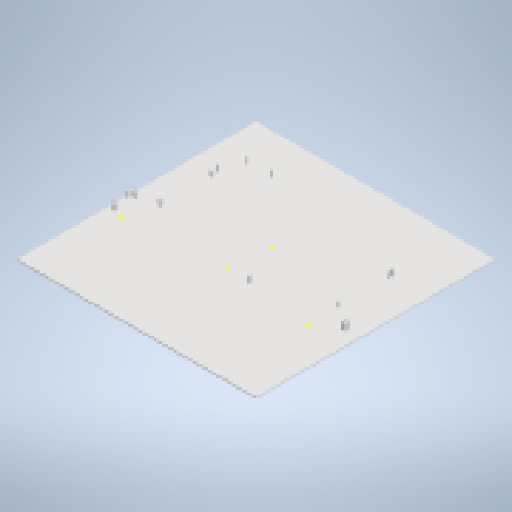
# Autodesk Inventor part: chassis
Saved by Autodesk Inventor 2025 (Build 290162010, 162A)
## iProperties
Created: 2025-12-11
Part Number: chassis
Material: Generic
Document SubType Name: Modeling
Designer: 200481997
Density: 1 g/cm^3
Appearance: Default
Author: 200481997
Autodesk Inventor part; units mm, degrees
ref_plane "YZ Plane" through (0, 0, 0) normal (1, 0, 0) x (0, 1, 0)
ref_plane "XZ Plane" through (0, 0, 0) normal (0, 1, 0) x (-1, 0, 0)
ref_plane "XY Plane" through (0, 0, 0) normal (0, 0, 1) x (1, 0, 0)
sketch "Sketch3" plane through (0, 0, 0) normal (0, 1, 0) x (-1, 0, 0)
  line L0 (-150, -128.5714) -> (150, -128.5714)
  line L1 (150, -128.5714) -> (150, 171.4286)
  line L2 (150, 171.4286) -> (-150, 171.4286)
  line L3 (-150, 171.4286) -> (-150, -128.5714)
  point P0 (0, 0)
  dimension "d80" = 300
  dimension "d81" = 300
  dimension "d82" = 150
  dimension "d83" = 128.5714
  constraints: 8 end point, 2 parallel, 1 horizontal, 1 perpendicular
  measures "d80" distance between parallel lines of L2 L0
  measures "d81" distance between parallel lines of L1 L3
  measures "d82" distance from line of point (0, 0) L3
  measures "d83" distance from line of point (0, 0) L0
extrude "Chassis base" add sketch "Sketch3" against normal blind 1.5875
sketch "Motherboard Mounting Holes" plane through (0, 0, 0) normal (0, 1, 0) x (-1, 0, 0)
  circle A0 centre (142.65, 56.4682) radius 1.15
  circle A1 centre (142.65, 56.4682) radius 2.5
  circle A2 centre (118.8, -41.6318) radius 2.05
  circle A3 centre (143.65, 30.0682) radius 1.15
  circle A4 centre (142.65, 56.4682) radius 2.5
  circle A5 centre (118.8, -41.6318) radius 0.7
  circle A6 centre (143.65, 30.0682) radius 2.5
  circle A7 centre (148.65, 51.0682) radius 1.1
  circle A8 centre (118.8, 22.3682) radius 0.7
  circle A9 centre (118.8, -41.6318) radius 2.05
  circle A10 centre (148.65, 34.0682) radius 1.1
  circle A11 centre (119.95, -50.0818) radius 1.25
  circle A12 centre (-102.85, -46.4318) radius 2
  circle A13 centre (-102.85, -46.4318) radius 0.9
  circle A14 centre (-103.35, 21.2682) radius 1.85
  circle A15 centre (-131, 40.4962) radius 4
  circle A16 centre (-103.35, 21.2682) radius 0.9
  circle A17 centre (-131, 40.4962) radius 1.35
  circle A18 centre (-103.35, -41.5818) radius 1.25
  circle A19 centre (-20.85, 50.0682) radius 0.9
  circle A20 centre (118.8, 22.3682) radius 2.05
  circle A21 centre (-20.85, 50.0682) radius 2
  circle A22 centre (118.8, -41.6318) radius 2.05
  circle A23 centre (142.65, 56.4682) radius 2.5
  circle A24 centre (118.8, -41.6318) radius 2.05
  circle A25 centre (148.65, 51.0682) radius 1.8
  circle A26 centre (148.65, 34.0682) radius 1.8
  line L0 (119.55, -51.2661) -> (119.55, -48.8975)
  line L1 (120.35, -48.8975) -> (120.35, -51.2661)
  line L2 (120.35, -51.6947) -> (119.55, -48.4689) construction
  line L3 (119.55, -51.6947) -> (120.35, -48.4689) construction
  line L4 (121.1343, -49.6818) -> (118.7657, -49.6818)
  line L5 (118.7657, -50.4818) -> (121.1343, -50.4818)
  line L6 (122.1914, -49.6818) -> (117.7086, -50.4818) construction
  line L7 (117.7086, -49.6818) -> (122.1914, -50.4818) construction
  line L8 (-103.75, -42.7661) -> (-103.75, -40.3975)
  line L9 (-102.95, -40.3975) -> (-102.95, -42.7661)
  line L10 (-102.95, -43.2946) -> (-103.75, -39.869) construction
  line L11 (-103.75, -43.2946) -> (-102.95, -39.869) construction
  line L12 (-102.1657, -41.1818) -> (-104.5343, -41.1818)
  line L13 (-104.5343, -41.9818) -> (-102.1657, -41.9818)
  line L14 (-101.5, -41.1818) -> (-105.2, -41.9818) construction
  line L15 (-105.2, -41.1818) -> (-101.5, -41.9818) construction
  point P0 (0, 0)
  point P1 (-102.95, -41.1818)
  point P2 (-103.75, -41.1818)
  point P3 (-103.75, -41.9818)
  point P4 (-102.95, -41.9818)
  point P5 (119.55, -50.4818)
  point P6 (120.35, -50.4818)
  point P7 (120.35, -49.6818)
  point P8 (119.55, -49.6818)
  dimension "d12" = 2.5
  dimension "d39" = 2.5
  dimension "d0" = 41.6318
  dimension "d1" = 118.8
  dimension "d2" = 8.45
  dimension "d3" = 1.15
  dimension "d8" = 102.85
  dimension "d9" = 46.4318
  dimension "d10" = 1.8
  dimension "d11" = 4
  dimension "d13" = 4.85
  dimension "d14" = 0.5
  dimension "d15" = 50.0682
  dimension "d16" = 20.85
  dimension "d17" = 1.8
  dimension "d18" = 4
  dimension "d19" = 103.35
  dimension "d20" = 21.2682
  dimension "d21" = 1.8
  dimension "d22" = 3.7
  dimension "d23" = 118.8
  dimension "d24" = 22.3682
  dimension "d25" = 1.4
  dimension "d26" = 4.1
  dimension "d27" = 143.65
  dimension "d28" = 30.0682
  dimension "d29" = 2.3
  dimension "d30" = 5
  dimension "d31" = 4
  dimension "d32" = 5
  dimension "d33" = 2.2
  dimension "d34" = 3.6
  dimension "d35" = 17
  dimension "d36" = 5.4
  dimension "d37" = 1.4
  dimension "d38" = 4.1
  dimension "d40" = 131
  dimension "d41" = 40.4962
  dimension "d42" = 6
  dimension "d52" = 8
  dimension "d53" = 2.7
  dimension "d66" = 0.8
  dimension "d67" = 0.8
  dimension "d68" = 0.8
  dimension "d69" = 0.8
  dimension "d71" = 0.4
  dimension "d72" = 0.4
  dimension "d73" = 0.4
  dimension "d74" = 0.4
  constraints: 32 end point, 25 centre point, 10 concentric, 8 midpoint, 4 equal radius, 4 parallel, 2 horizontal, 1 vertical alignment, 20 other
  measures "d0" vertical distance of point (0, 0) A2.centre
  measures "d1" horizontal distance of point (0, 0) A2.centre
  measures "d2" vertical distance of A2.centre point (119.95, -50.082)
  measures "d3" horizontal distance of point (119.95, -50.082) A2.centre
  measures "d8" horizontal distance of point (0, 0) A12.centre
  measures "d9" vertical distance of point (0, 0) A12.centre
  measures "d10" diameter of A13
  measures "d11" diameter of A12
  measures "d13" vertical distance of point (-103.35, -41.582) A12.centre
  measures "d14" horizontal distance of A12.centre point (-103.35, -41.582)
  measures "d15" vertical distance of point (0, 0) A19.centre
  measures "d16" horizontal distance of point (0, 0) A19.centre
  measures "d17" diameter of A19
  measures "d18" diameter of A21
  measures "d19" horizontal distance of point (0, 0) A14.centre
  measures "d20" vertical distance of A14.centre point (0, 0)
  measures "d21" diameter of A16
  measures "d22" diameter of A14
  measures "d23" horizontal distance of point (0, 0) A8.centre
  measures "d24" vertical distance of point (0, 0) A8.centre
  measures "d25" diameter of A8
  measures "d26" diameter of A20
  measures "d27" horizontal distance of point (0, 0) A3.centre
  measures "d28" vertical distance of point (0, 0) A3.centre
  measures "d29" diameter of A3
  measures "d30" diameter of A6
  measures "d31" vertical distance of A3.centre A10.centre
  measures "d32" horizontal distance of A3.centre A10.centre
  measures "d33" diameter of A10
  measures "d34" diameter of A26
  measures "d35" distance of A7.centre A26.centre
  measures "d36" vertical distance of A7.centre A0.centre
  measures "d37" diameter of A5
  measures "d38" diameter of A2
  measures "d40" horizontal distance of point (0, 0) A15.centre
  measures "d41" vertical distance of point (0, 0) A15.centre
  measures "d42" horizontal distance of A7.centre A0.centre
  measures "d52" diameter of A15
  measures "d53" diameter of A17
  measures "d66" distance between parallel lines of L4 L5
  measures "d67" distance between parallel lines of L0 L1
  measures "d68" distance between parallel lines of L12 L13
  measures "d69" distance between parallel lines of L8 L9
  measures "d71" distance from line of point (-103.35, -41.582) L12
  measures "d72" distance from line of point (-103.35, -41.582) L9
  measures "d73" distance from line of point (119.95, -50.082) L5
  measures "d74" distance from line of L0 point (119.95, -50.082)
sketch "DP adapter Mounting Holes" plane through (0, 0, 0) normal (0, 1, 0) x (1, 0, 0)
  circle A0 centre (-109.8518, 77.3373) radius 1.27
  circle A1 centre (-79.6718, 77.3373) radius 1.27
  circle A2 centre (-109.8518, 77.3373) radius 0.7
  circle A3 centre (-79.6718, 77.3373) radius 0.7
  point P0 (0, 0)
  dimension "d45" = 2.54
  dimension "d46" = 30.18
  dimension "d47" = 1.4
  constraints: 4 centre point, 2 coincident, 2 equal radius, 1 horizontal alignment
  measures "d45" diameter of A0
  measures "d46" distance of A0.centre A1.centre
  measures "d47" diameter of A2
extrude "Motherboard Mounting Extrusions" add sketch "Motherboard Mounting Holes" along normal blind 7.1 contours A2 | A12 | A14 | A20 | A21
extrude "Motherboard Support Extrusions" add sketch "Motherboard Mounting Holes" along normal blind 7.75 contours A11 L5 L1 L4 | L1 L4 L0 A11 | L1 L5 L0 L4 | A11 L0 L5 L1 | L0 L5 A11 L4 | A18 L13 L9 L12 | L9 L12 L8 A18 | L9 L13 L8 L12 | A18 L8 L13 L9 | L8 L13 A18 L12
chamfer "Motherboard Support Chamfer" distance 0.3556 angle 45 8 edges at (103.35, 7.75, -42.8318) (104.6, 7.75, -41.5818) (103.35, 7.75, -40.3318) (102.1, 7.75, -41.5818) (-118.7, 7.75, -50.0818) (-119.95, 7.75, -51.3318) (-121.2, 7.75, -50.0818) (-119.95, 7.75, -48.8318)
extrude "Headphone Mounting Extrusions" add sketch "Motherboard Mounting Holes" along normal blind 7.9 contours A1 | A6
extrude "Headphone Support Base" add sketch "Motherboard Mounting Holes" along normal blind 5.4 contours A7 | A10 | A25 | A26
extrude "Headphone Support" add sketch "Motherboard Mounting Holes" along normal blind 2.1 from surface at 5.4 contours A7 | A10
fillet "Round Headphone Support" radius 0.381 2 edges at (-147.55, 7.5, 34.0682) (-147.55, 7.5, 51.0682)
extrude "Wifi Card Mounting Extrusion" add sketch "Motherboard Mounting Holes" along normal blind 8.685 contours A15
chamfer "Wifi Card Mount Chamfer" distance 1.143 angle 45 1 edges at (135, 8.685, 40.4962)
extrude "DP adapter Mouting Extrusions" add sketch "DP adapter Mounting Holes" along normal blind 7.62
sketch "Sketch6" plane through (0, 0, 0) normal (0, 1, 0) x (1, 0, 0)
  circle A0 centre (-128.9436, -60.8279) radius 0.8509
  circle A1 centre (-128.9436, -60.8279) radius 1.0033
  circle A2 centre (-6.9474, -49.5503) radius 1.0033
  circle A3 centre (-6.9474, -49.5503) radius 0.8509
  circle A4 centre (69.7908, -38.859) radius 0.8509
  circle A5 centre (69.7908, -38.859) radius 1.0033
  point P0 (0, 0)
  dimension "d86" = 1.7018
  dimension "d87" = 2.0066
  dimension "d88" = 121.9962
  dimension "d89" = 11.2776
  constraints: 6 centre point, 4 equal radius, 3 coincident
  measures "d86" diameter of A0
  measures "d87" diameter of A1
  measures "d88" horizontal distance of A0.centre A2.centre
  measures "d89" vertical distance of A0.centre A2.centre
body "Solid1"
